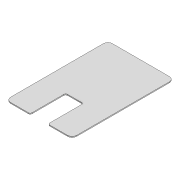
# Autodesk Inventor part: led_ring_cover
Saved by Autodesk Inventor 2020 (Build 240168000, 168)
## iProperties
Created: 2020-05-07
Part Number: led_ring_cover
Material: Generic
Document SubType Name: Modeling
Designer: User
Density: 1 g/cm^3
Appearance: Default
Author: User
Autodesk Inventor part; units mm, degrees
ref_plane "YZ Plane" through (0, 0, 0) normal (1, 0, 0) x (0, 1, 0)
ref_plane "XZ Plane" through (0, 0, 0) normal (0, 1, 0) x (-1, 0, 0)
ref_plane "XY Plane" through (0, 0, 0) normal (0, 0, 1) x (1, 0, 0)
sketch "Sketch1" plane through (0, 0, 0) normal (0, 1, 0) x (-1, 0, 0)
  line L0 (-27.94, -43.053) -> (27.94, -43.053)
  line L1 (27.94, -43.053) -> (27.94, 43.053)
  line L2 (27.94, 43.053) -> (-27.94, 43.053)
  line L3 (-27.94, 43.053) -> (-27.94, -43.053)
  line L4 (-27.94, -43.053) -> (27.94, 43.053) construction
  line L5 (27.94, -43.053) -> (-27.94, 43.053) construction
  point P0 (0, 0)
  dimension "d0" = 86.106
  dimension "d1" = 55.88
  constraints: 12 end point, 2 midpoint, 2 parallel, 1 horizontal, 1 perpendicular
  measures "d0" distance of L0.end L1.end
  measures "d1" distance of L1.end L2.end
extrude "Extrusion1" add sketch "Sketch1" along normal blind 0.8
fillet "Fillet1" radius 3.9688 4 edges at (27.94, 0.4, 43.053) (27.94, 0.4, -43.053) (-27.94, 0.4, -43.053) (-27.94, 0.4, 43.053)
sketch "Sketch2" plane through (0, 0.8, 0) normal (0, 1, 0) x (1, 0, 0)
  line L0 (7.5, -73.053) -> (-7.5, -73.053)
  line L1 (-7.5, -73.053) -> (-7.5, -13.053)
  line L2 (-7.5, -13.053) -> (7.5, -13.053)
  line L3 (7.5, -13.053) -> (7.5, -73.053)
  line L4 (-23.9712, -43.053) -> (23.9713, -43.053) projected
  line L5 (7.5, -73.053) -> (-7.5, -13.053) construction
  line L6 (-7.5, -73.053) -> (7.5, -13.053) construction
  point P0 (0, 0)
  point P1 (0, -43.053)
  point P2 (-7.5, -43.053)
  point P3 (7.5, -43.053)
  dimension "d5" = 15
  dimension "d6" = 60
  constraints: 12 end point, 3 midpoint, 2 parallel, 1 horizontal, 1 perpendicular
  measures "d5" distance of L1.end L2.end
  measures "d6" distance of L0.end L1.end
extrude "Extrusion2" cut sketch "Sketch2" against normal blind 25.4 contours L4 L1 L2 L3
fillet "Fillet2" radius 1.5875 4 edges at (-7.5, 0.4, 13.053) (7.5, 0.4, 13.053) (-7.5, 0.4, 43.053) (7.5, 0.4, 43.053)
body "Solid1"
